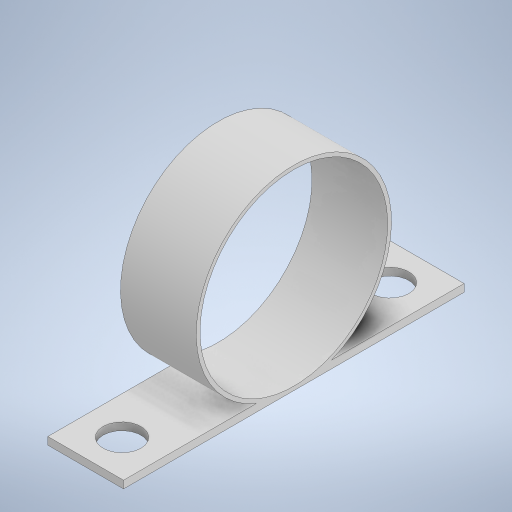
# Autodesk Inventor part: apoiom
Saved by Autodesk Inventor 2024 (Build 280153020, 153B)
## iProperties
Created: 2023-06-05
Part Number: apoiom
Material: Genérico
Document SubType Name: Modeling
Designer: victo
Density: 1 g/cm^3
Appearance: Padrão
Author: victo
Autodesk Inventor part; units mm, degrees
ref_plane "YZ Plane" through (0, 0, 0) normal (1, 0, 0) x (0, 1, 0)
ref_plane "XZ Plane" through (0, 0, 0) normal (0, 1, 0) x (-1, 0, 0)
ref_plane "XY Plane" through (0, 0, 0) normal (0, 0, 1) x (1, 0, 0)
sketch "Esboço1" plane through (0, 0, 0) normal (1, 0, 0) x (0, 1, 0)
  arc A0 (-11.9, -4.98) -> (-11.9, 4.98) centre (0, 0) ccw
  circle A1 centre (0, 0) radius 12.4
  line L0 (-12.9, 0) -> (-12.9, 22.5)
  line L1 (-12.9, 22.5) -> (-11.9, 22.5)
  line L2 (-11.9, 22.5) -> (-11.9, 4.98)
  line L3 (-12.9, 0) -> (-12.9, -22.5)
  line L4 (-12.9, -22.5) -> (-11.9, -22.5)
  line L5 (-11.9, -4.98) -> (-11.9, -22.5)
  point P0 (-11.9, 4.98)
  dimension "d57" = 25.8
  dimension "d58" = 24.8
  dimension "d72" = 22.5
  dimension "d73" = 22.5
  constraints: 12 end point, 4 vertical, 2 centre point, 2 point on circle, 1 coincident
  measures "d57" diameter of A0
  measures "d58" diameter of A1
  measures "d72" distance of L0.start L0.end
  measures "d73" distance of L0.start L3.end
extrude "Extrusão8" add sketch "Esboço1" against normal blind 10
sketch "Esboço7" plane through (0, -11.9, 22.5) normal (0, 1, 0) x (1, 0, 0)
  line L0 (0, 35.4) -> (-10, 35.4) projected
  line L1 (0, 0) -> (-10, 0) projected
  circle A0 centre (-5, 4.8) radius 2.5
  circle A1 centre (-5, 40.2) radius 2.5
  point P0 (0, 22.5)
  dimension "d78" = 5
  dimension "d79" = 5
  constraints: 2 centre point
  measures "d78" diameter of A0
  measures "d79" diameter of A1
extrude "Extrusão9" cut sketch "Esboço7" against normal up to next
